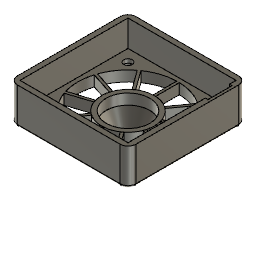
40x10_turbine_fan_cover (Autodesk Fusion 360 design; units mm, degrees)
part number: 2026-02-26-21-48-31-019
Autodesk Fusion 360 part; units mm, degrees
sketch "Skizze1" plane through (0, 0, 0) normal (0, 0, 1) x (1, 0, 0)
  line L0 (20.5, -20.5) -> (-20.5, -20.5)
  line L1 (-20.5, -20.5) -> (-20.5, 20.5)
  line L2 (-20.5, 20.5) -> (20.5, 20.5)
  line L3 (20.5, 20.5) -> (20.5, -20.5)
  line L4 (20.5, -20.5) -> (-20.5, 20.5) construction
  line L5 (-20.5, -20.5) -> (20.5, 20.5) construction
  circle A0 centre (-16.0004, 16.0004) radius 1.6
  circle A1 centre (-16.0004, 16.0004) radius 2.75
  line L6 (-22.5, -22.5) -> (-22.5, 22.5)
  line L7 (-22.5, 22.5) -> (22.5, 22.5)
  line L8 (22.5, 22.5) -> (22.5, -22.5)
  line L9 (22.5, -22.5) -> (-22.5, -22.5)
  dimension "d1" = 41
  dimension "d2" = 41
  dimension "d3" = 3.2
  dimension "d4" = 5.5
  dimension "d5" = -2
  constraint horizontal L0
  constraint perpendicular L0 L1
  constraint parallel L0 L2
  constraint parallel L1 L3
  constraint coincident L4 origin
  constraint coincident L5 origin
  constraint coincident L4 A0.centre
  constraint concentric A0 A1
  measures "d1" distance of L1.end L2.end
  measures "d2" distance of L0.end L1.end
  measures "d3" diameter of A0
  measures "d4" diameter of A1
other "Grundnetzelement1"
extrude "Extrusion1" add sketch "Skizze1" along normal blind 4 contours L0 L1 L2 L3 | A0 | A1 makes body 1
extrude "Extrusion2" add sketch "Skizze1" along normal blind 14 separate body contours L6 L7 L8 L9 makes body 2
extrude "Extrusion3" cut sketch "Skizze1" along normal blind 4 contours A0 bodies 1
extrude "Extrusion4" cut sketch "Skizze1" along normal blind 2.5 contours A1 bodies 1
mirror "Spiegeln1" about plane through (0, 0, 0) normal (1, 0, 0) of "Extrusion3", "Extrusion4"
mirror "Spiegeln2" about plane through (0, 0, 0) normal (0, 1, 0) of "Extrusion3", "Extrusion4"
mirror "Spiegeln3" about plane through (0, 0, 0) normal (1, 0, 0) of "Spiegeln2"
fillet "Abrundung1" radius 3 4 edges at (22.5, 22.5, 7) (22.5, -22.5, 7) (-22.5, 22.5, 7) (-22.5, -22.5, 7) on bodies 2
fillet "Abrundung2" radius 1 8 edges at (21.6213, 21.6213, 0) (22.5, 0, 0) (21.6213, -21.6213, 0) (0, -22.5, 0) (-21.6213, -21.6213, 0) (-22.5, 0, 0) (-21.6213, 21.6213, 0) (0, 22.5, 0) on bodies 2
sketch "Skizze2" plane through (0, 0, 0) normal (0, 0, -1) x (1, 0, 0)
  circle A0 centre (16.0004, 16.0004) radius 2.75
  circle A1 centre (-16.0004, 16.0004) radius 2.75
  circle A2 centre (16.0004, -16.0004) radius 2.75
  circle A3 centre (-16.0004, -16.0004) radius 2.75
  line L0 (-20.5, -20.5) -> (20.5, -20.5)
  line L1 (20.5, -20.5) -> (20.5, 20.5)
  line L2 (20.5, 20.5) -> (-20.5, 20.5)
  line L3 (-20.5, 20.5) -> (-20.5, -20.5)
  circle A4 centre (0, 0) radius 19
  circle A5 centre (0, 0) radius 10
  line L4 (0, 19) -> (0, 10)
  line L5 (0.5, 10) -> (-0.5, 10)
  line L6 (-0.5, 10) -> (-0.5, 19)
  line L7 (-0.5, 19) -> (0.5, 19)
  line L8 (0.5, 19) -> (0.5, 10)
  line L9 (0.5, 10) -> (-0.5, 19) construction
  line L10 (-0.5, 10) -> (0.5, 19) construction
  line L11 (-6.2824, 7.7963) -> (-11.5724, 15.0774)
  line L12 (-11.5724, 15.0774) -> (-10.7634, 15.6652)
  line L13 (-5.4733, 8.3841) -> (-6.2824, 7.7963)
  line L14 (-10.7634, 15.6652) -> (-5.4733, 8.3841)
  line L15 (-9.6651, 2.6146) -> (-18.2246, 5.3958)
  line L16 (-18.2246, 5.3958) -> (-17.9156, 6.3469)
  line L17 (-9.3561, 3.5657) -> (-9.6651, 2.6146)
  line L18 (-17.9156, 6.3469) -> (-9.3561, 3.5657)
  line L19 (-9.3561, -3.5657) -> (-17.9156, -6.3469)
  line L20 (-17.9156, -6.3469) -> (-18.2246, -5.3958)
  line L21 (-9.6651, -2.6146) -> (-9.3561, -3.5657)
  line L22 (-18.2246, -5.3958) -> (-9.6651, -2.6146)
  line L23 (-5.4733, -8.3841) -> (-10.7634, -15.6652)
  line L24 (-10.7634, -15.6652) -> (-11.5724, -15.0774)
  line L25 (-6.2824, -7.7963) -> (-5.4733, -8.3841)
  line L26 (-11.5724, -15.0774) -> (-6.2824, -7.7963)
  line L27 (0.5, -10) -> (0.5, -19)
  line L28 (0.5, -19) -> (-0.5, -19)
  line L29 (-0.5, -10) -> (0.5, -10)
  line L30 (-0.5, -19) -> (-0.5, -10)
  line L31 (6.2824, -7.7963) -> (11.5724, -15.0774)
  line L32 (11.5724, -15.0774) -> (10.7634, -15.6652)
  line L33 (5.4733, -8.3841) -> (6.2824, -7.7963)
  line L34 (10.7634, -15.6652) -> (5.4733, -8.3841)
  line L35 (9.6651, -2.6146) -> (18.2246, -5.3958)
  line L36 (18.2246, -5.3958) -> (17.9156, -6.3469)
  line L37 (9.3561, -3.5657) -> (9.6651, -2.6146)
  line L38 (17.9156, -6.3469) -> (9.3561, -3.5657)
  line L39 (9.3561, 3.5657) -> (17.9156, 6.3469)
  line L40 (17.9156, 6.3469) -> (18.2246, 5.3958)
  line L41 (9.6651, 2.6146) -> (9.3561, 3.5657)
  line L42 (18.2246, 5.3958) -> (9.6651, 2.6146)
  line L43 (5.4733, 8.3841) -> (10.7634, 15.6652)
  line L44 (10.7634, 15.6652) -> (11.5724, 15.0774)
  line L45 (6.2824, 7.7963) -> (5.4733, 8.3841)
  line L46 (11.5724, 15.0774) -> (6.2824, 7.7963)
  point P0 (0, 14.5)
  point P1 (0, 14.5)
  dimension "d24" = 38
  dimension "d25" = 20
  dimension "d26" = 1
  dimension "d27" = 9
  dimension "d29" = 360
  constraint coincident A4.centre A5.centre
  constraint concentric A4 A5
  constraint coincident A4 L4.start
  constraint coincident A5 L4.end
  constraint vertical L4
  constraint midpoint L4 P1
  constraint horizontal L5
  constraint perpendicular L5 L6
  constraint parallel L5 L7
  constraint parallel L6 L8
  constraint coincident L9 P1
  constraint coincident L10 P1
  constraint coincident P1 P0
  measures "d24" diameter of A4
  measures "d25" diameter of A5
  measures "d26" distance of L6.end L7.end
  measures "d27" distance of L5.end L6.end
ref_plane "Arbeitsebene1" through (0, 0, -4.3674) normal (0, 1, 0) x (0, 0, -1)
sketch "Skizze3" plane through (0, 0, 0) normal (0, 1, 0) x (1, 0, 0)
  circle A0 through (10, 0, 0) (-5, 0, 8.6603) (-5, 0, -8.6603)
  line L0 (10, 0) -> (0, 17.3205)
  line L1 (0, 17.3205) -> (0, 0)
  line L2 (0, 0) -> (10, 0)
  line L3 (0, 14.3205) -> (8.2679, 0)
  line L4 (0, -6.7054) -> (0, 15.4402)
  dimension "d31" = 20
  dimension "d36" = 1.5
  constraint coincident L1.end L2.start
  constraint horizontal L2
  constraint coincident L1 L3.start
  constraint coincident L2 L3.end
  constraint parallel L0 L3
  constraint coincident L0.end L4
  measures "d31" distance of L0.start L0.end
  measures "d36" distance of L0 L3
revolve "Drehen1" add sketch "Skizze3" angle 360 about axis through (0, 0, -17.3205) along (0, 0, 1) separate body makes body 3
extrude "Extrusion5" cut sketch "Skizze2" against normal blind 4 contours A4 A5 L35 L37 L41 L42 | A4 A5 L39 L41 L45 L46 | A4 A5 L31 L33 L37 L38 | A4 A5 L5 L8 L43 L45 | A4 A5 L27 L29 L33 L34 | A4 A5 L5 L6 L13 L14 | A4 A5 L23 L25 L29 L30 | A4 A5 L11 L13 L17 L18 | A4 A5 L19 L21 L25 L26 | A4 A5 L15 L17 L21 L22 bodies 1
revolve "Drehen4" cut sketch "Skizze3" angle 360 about axis through (0, 0, -17.3205) along (0, 0, 1) contours L1 L2 L3 L4 bodies 3
sketch "Skizze4" plane through (0, 0, 0) normal (0, 0, -1) x (1, 0, 0)
  circle A0 centre (0, 0) radius 8.2679
  point P0 (8.2679, 0)
  constraint coincident A0.centre origin
  constraint coincident A0 P0
extrude "Extrusion6" cut sketch "Skizze4" against normal blind 4 bodies 1
sketch "Skizze5" plane through (20.5, 0, 0) normal (-1, 0, 0) x (0, -1, 0)
  line L0 (-20.5, 0) -> (20.5, 0)
  line L1 (20.5, 0) -> (20.5, 14)
  line L2 (20.5, 14) -> (-20.5, 14)
  line L3 (-20.5, 14) -> (-20.5, 0)
  line L4 (-8.905, 5.7893) -> (-18, 5.7893)
  line L5 (-18, 5.7893) -> (-18, 14)
  line L6 (-18, 14) -> (-8.905, 14)
  line L7 (-8.905, 14) -> (-8.905, 5.7893)
  constraint horizontal L4
  constraint vertical L5
  constraint horizontal L6
  constraint vertical L7
  constraint coincident L2 L5.end
extrude "Extrusion7" cut sketch "Skizze5" against normal blind 1 contours L2 L4 L5 L6 L7 bodies 2
